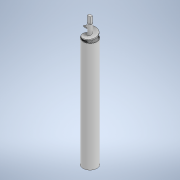
# Autodesk Inventor part: Arkimedes skruv
Saved by Autodesk Inventor 2021 (Build 250183000, 183)
## iProperties
Created: 2024-12-11
Part Number: Arkimedes skruv
Material: Generic
Document SubType Name: Modeling
Designer: 24lucsil
Density: 1 g/cm^3
Appearance: Default
Author: 24lucsil
Autodesk Inventor part; units mm, degrees
ref_plane "YZ Plane" through (0, 0, 0) normal (1, 0, 0) x (0, 1, 0)
ref_plane "XZ Plane" through (0, 0, 0) normal (0, 1, 0) x (-1, 0, 0)
ref_plane "XY Plane" through (0, 0, 0) normal (0, 0, 1) x (1, 0, 0)
sketch "Sketch1" plane through (0, 0, 0) normal (0, 1, 0) x (-1, 0, 0)
  circle A0 centre (0, 0) radius 65.1659
  circle A1 centre (0, 0) radius 3
  dimension "d0" = 6
  constraints: 2 centre point, 2 coincident
  measures "d0" diameter of A1
extrude "Extrusion1" add sketch "Sketch1" along normal blind 200 contours A1
sketch "Sketch2" plane through (0, 0, 0) normal (0, 0, 1) x (1, 0, 0)
  line L0 (3, 0) -> (-3, 0) projected
  line L1 (-3, 0) -> (-10, 0)
  line L2 (-10, 0) -> (-10, 1.5)
  line L3 (-10, 1.5) -> (-3, 1.5)
  line L4 (-3, 1.5) -> (-3, 0)
  point P0 (0, 0)
  dimension "d3" = 7
  dimension "d4" = 1.5
  constraints: 8 end point, 2 parallel, 1 horizontal, 1 perpendicular
  measures "d3" distance of L0.end L1.end
  measures "d4" distance of L1.end L2.end
coil "Coil1" sketch "Sketch2" operation add axis through (0, -10, 0) along (0, 1, 0) pitch 10 turns 18 hand right
sketch "Sketch3" plane through (0, 0, 0) normal (0, -1, 0) x (1, 0, 0)
  circle A0 centre (0, 0) radius 10
  circle A1 centre (0, 0) radius 10.75
  dimension "d13" = 20
  dimension "d14" = 21.5
  constraints: 2 centre point, 2 coincident
  measures "d13" diameter of A0
  measures "d14" diameter of A1
extrude "Extrusion2" add sketch "Sketch3" against normal blind 170
sketch "Sketch6" plane through (0, 200, 0) normal (0, 1, 0) x (1, 0, 0)
  circle A0 centre (0, 0) radius 2.75
  line L0 (0, -2.75) -> (0, -1.75)
  line L1 (0, 2.75) -> (0, 1.75)
  line L2 (0, 1.75) -> (0, -1.75)
  line L3 (2.1213, 1.75) -> (-2.1213, 1.75)
  line L4 (2.1213, -1.75) -> (-2.1213, -1.75)
  circle A1 centre (0, 0) radius 3
  dimension "d31" = 5.5
  dimension "d32" = 1
  dimension "d33" = 1
  dimension "d34" = 3.5
  constraints: 10 end point, 6 point on circle, 3 vertical, 2 centre point, 2 coincident, 2 horizontal
  measures "d31" diameter of A0
  measures "d32" distance of L0.start L0.end
  measures "d33" distance of L1.start L1.end
  measures "d34" distance between parallel lines of L4 L3
extrude "Extrusion3" cut sketch "Sketch6" against normal blind 10 contours L3 L1 A0 | A0 L0 L4 | L1 L3 A0 | A0 L4 L0 | A1
body "Solid1"
